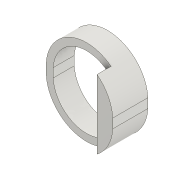
# Autodesk Inventor part: Midlle inner console for tilting head
Saved by Autodesk Inventor 2020.3 (Build 243373010, 373A)
## iProperties
Created: 2021-05-15
Part Number: Midlle inner console for tilting head
Material: Steel AISI 4620
Document SubType Name: Modeling
Designer: marti
Density: 7.85 g/cm^3
Appearance: Steel
Author: marti
Autodesk Inventor part; units mm, degrees
ref_plane "YZ Plane" through (0, 0, 0) normal (1, 0, 0) x (0, 1, 0)
ref_plane "XZ Plane" through (0, 0, 0) normal (0, 1, 0) x (-1, 0, 0)
ref_plane "XY Plane" through (0, 0, 0) normal (0, 0, 1) x (1, 0, 0)
sketch "Sketch1" plane through (0, 0, 0) normal (0, 0, 1) x (1, 0, 0)
  arc A0 (-27.9541, -8.4837) -> (27.9541, -8.4837) centre (0, -1.7656) ccw
  arc A1 (-28.7072, -3.3345) -> (28.7072, -3.3345) centre (0, -1.7656) ccw
  line L0 (28.7072, 3.3345) -> (28.7072, -3.3345)
  arc A2 (28.7072, 3.3345) -> (-28.7072, 3.3345) centre (0, 1.7656) ccw
  line L1 (-28.7072, -3.3345) -> (-28.7072, 3.3345)
  arc A3 (23.7072, 3.1915) -> (-23.7072, 3.1915) centre (0, 1.7656) ccw
  line L2 (23.7072, 3.1915) -> (23.7072, -3.1915)
  arc A4 (-23.7072, -3.1915) -> (23.7072, -3.1915) centre (0, -1.7656) ccw
  line L3 (-23.7072, -3.1915) -> (-23.7072, 3.1915)
  point P0 (0, 0)
  point P1 (0, 0)
  dimension "d0" = 5
  constraints: 10 point on circle, 8 end point, 5 centre point, 3 other
  measures "d0" radial gap between concentric circles of A2 A3
extrude "Extrusion1" add sketch "Sketch1" along normal mid plane 15
sketch "Sketch3" plane through (0, 0, 7.5) normal (0, 0, 1) x (1, 0, 0)
  line L0 (17.5002, -24.5758) -> (17.5002, 24.5758)
  line L1 (23.7072, 3.1915) -> (23.7072, -3.1915) projected
  arc A0 (-23.7072, -3.1915) -> (23.7072, -3.1915) centre (0, -1.7656) ccw projected
  arc A1 (23.7072, 3.1915) -> (-23.7072, 3.1915) centre (0, 1.7656) ccw projected
  arc A2 (28.7072, 3.3345) -> (-28.7072, 3.3345) centre (0, 1.7656) ccw projected
  line L2 (-28.7072, 3.3345) -> (-28.7072, -3.3345) projected
  arc A3 (-28.7072, -3.3345) -> (28.7072, -3.3345) centre (0, -1.7656) ccw projected
  line L3 (28.7072, -3.3345) -> (28.7072, 3.3345) projected
  line L4 (-23.7072, -3.1915) -> (-23.7072, 3.1915) projected
  arc A4 (23.7072, 3.1915) -> (-23.7072, 3.1915) centre (0, 1.7656) ccw projected
  line L5 (23.7072, 3.1915) -> (23.7072, -3.1915) projected
  arc A5 (-23.7072, -3.1915) -> (23.7072, -3.1915) centre (0, -1.7656) ccw projected
  point P0 (0, 0)
  dimension "d3" = 6.207
  constraints: 2 end point, 2 point on circle, 1 vertical
  measures "d3" distance between parallel lines of L0 L1
extrude "Extrusion2" add sketch "Sketch3" along normal blind 10 contours L0 A0 L1 A1 A2 L3 A3 | L0 A1 L1 A0
fillet "Fillet1" radius 2 3 edges at (21.8638, 11.0413, 7.5) (23.7072, 0, 7.5) (21.8638, -11.0413, 7.5)
body "Solid1"
